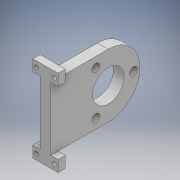
# Autodesk Inventor part: Slipring_mount
Saved by Autodesk Inventor 2017 (Build 210142000, 142)
## iProperties
Created: 2017-04-29
Part Number: Slipring_mount
Material: Generic
Document SubType Name: Modeling
Designer: s4321966
Density: 1 g/cm^3
Appearance: Default
Author: s4321966
Autodesk Inventor part; units mm, degrees
ref_plane "YZ Plane" through (0, 0, 0) normal (1, 0, 0) x (0, 1, 0)
ref_plane "XZ Plane" through (0, 0, 0) normal (0, 1, 0) x (-1, 0, 0)
ref_plane "XY Plane" through (0, 0, 0) normal (0, 0, 1) x (1, 0, 0)
sketch "Sketch1" plane through (0, 0, 0) normal (1, 0, 0) x (0, 1, 0)
  circle A0 centre (0, 0) radius 11
  circle A1 centre (0, 0) radius 22
  circle A2 centre (0, 0) radius 17.5
  circle A3 centre (17.5, 0) radius 2.75
  circle A4 centre (-8.75, 15.1554) radius 2.75
  circle A5 centre (-8.75, -15.1554) radius 2.75
  dimension "d2" = 35
  dimension "d0" = 22
  dimension "d1" = 44
  dimension "d3" = 5.5
  dimension "d6" = 360
  constraints: 5 centre point, 3 coincident, 1 horizontal alignment, 9 other
  measures "d0" diameter of A0
  measures "d1" diameter of A1
  measures "d3" diameter of A3
extrude "Extrusion1" add sketch "Sketch1" along normal blind 7.5 contours A1 | A3 A2 A5 A4
sketch "Sketch2" plane through (7.5, 0, 0) normal (1, 0, 0) x (0, 0, -1)
  arc A0 (2.7415, 17.2839) -> (-2.7415, 17.2839) centre (0, 0) ccw projected
  circle A1 centre (0, 0) radius 17.5
  circle A2 centre (0, 17.5) radius 2.75
  circle A3 centre (-15.1554, -8.75) radius 2.75
  circle A4 centre (15.1554, -8.75) radius 2.75
  dimension "d10" = 35
  dimension "d11" = 5.5
  dimension "d14" = 360
  constraints: 3 centre point, 1 coincident, 1 vertical alignment, 9 other
  measures "d11" diameter of A2
extrude "Extrusion2" cut sketch "Sketch2" against normal blind 10 contours A2 A0 | A0 A2 | A3 A1 | A1 A3 | A4 A1 | A1 A4
sketch "Sketch3" plane through (7.5, 0, 0) normal (1, 0, 0) x (0, 0, -1)
  line L0 (0, 0) -> (0, -40)
  line L1 (0, 0) -> (40, 0) construction
  line L2 (0, -40) -> (50, -40)
  line L3 (0, -40) -> (25, -40)
  line L4 (25, -40) -> (25, -35)
  line L5 (25, -35) -> (0, -35)
  line L6 (0, -35) -> (0, -40)
  line L7 (0, -35) -> (30, -35)
  line L8 (30, -35) -> (30, -40)
  line L9 (30, -40) -> (0, -40)
  line L10 (0, -40) -> (0, -35)
  line L11 (30, -40) -> (-30, -40)
  line L12 (-30, -40) -> (-30, -35)
  line L13 (-30, -35) -> (30, -35)
  line L14 (30, -35) -> (30, -40)
  circle A0 centre (0, 0) radius 22 projected
  line L15 (25, -40) -> (-22, -40)
  line L16 (-22, -40) -> (-22, 0)
  line L17 (-22, 0) -> (25, 0)
  line L18 (22, 0) -> (-22, 0)
  line L19 (-22, 0) -> (-22, -40)
  line L20 (-22, -40) -> (22, -40)
  line L21 (22, -40) -> (22, 0)
  line L22 (30, -35) -> (22, -35)
  line L23 (22, -35) -> (22, -40)
  line L24 (22, -40) -> (30, -40)
  line L25 (30, -40) -> (30, -35)
  line L26 (-30, -35) -> (-22, -35)
  line L27 (-22, -35) -> (-22, -40)
  line L28 (-22, -40) -> (-30, -40)
  line L29 (-30, -40) -> (-30, -35)
  dimension "d18" = 40
  dimension "d19" = 90
  dimension "d20" = 50
  dimension "d21" = 25
  dimension "d22" = 5
  dimension "d23" = 30
  dimension "d24" = 5
  dimension "d25" = 60
  dimension "d26" = 5
  constraints: 60 end point, 13 parallel, 9 perpendicular, 8 horizontal, 2 point on circle, 1 point on line, 1 vertical
  measures "d18" distance of L0.start L0.end
  measures "d19" angle of L0 L1
  measures "d20" distance of L0.end L2.end
  measures "d21" distance of L5.end L4.end
  measures "d22" distance of L4.end L3.end
  measures "d23" distance of L8.end L9.end
  measures "d24" distance of L7.end L8.end
  measures "d25" distance of L12.end L13.end
  measures "d26" distance of L11.end L12.end
extrude "Extrusion3" add sketch "Sketch3" against normal blind 7.5 contours L5 L21 L2 L0 | L13 L16 A0 L0 | L0 A0 L21 L5 | L0 L11 L16 L13 | L5 L4 L2 L21 | L16 L11 L12 L13 | L7 L8 L2 L4
sketch "Sketch5" plane through (7.5, 0, 0) normal (1, 0, 0) x (0, 0, -1)
  line L0 (30, -35) -> (30, -40) projected
  line L1 (22, -35) -> (30, -35) projected
  line L2 (30, -40) -> (22, -40)
  line L3 (22, -40) -> (22, -35)
  line L4 (22, -35) -> (30, -35)
  line L5 (30, -35) -> (30, -40)
  line L6 (-30, -35) -> (-30, -40) projected
  line L7 (-30, -40) -> (-22, -40)
  line L8 (-22, -40) -> (-22, -35)
  line L9 (-22, -35) -> (-30, -35)
  line L10 (-30, -35) -> (-30, -40)
  point P0 (0, 0)
  constraints: 16 end point, 4 parallel, 2 horizontal, 2 perpendicular
extrude "Extrusion5" add sketch "Sketch5" along normal blind 5 and the other way blind 12.5
sketch "Sketch6" plane through (-5, -35, -30) normal (0, 1, 0) x (1, 0, 0)
  line L0 (0, -8) -> (5, -8) projected
  line L1 (0, 0) -> (17.5, 0) projected
  line L2 (5, -8) -> (0, 0)
  line L3 (0, 0) -> (17.5, 0)
  line L4 (12.5, -8) -> (5, -8) projected
  line L5 (17.5, 0) -> (12.5, -8)
  line L6 (0, -52) -> (5, -52) projected
  line L7 (12.5, -8) -> (5, -52)
  line L8 (17.5, -60) -> (0, -60) projected
  line L9 (5, -52) -> (0, -60)
  line L10 (0, -60) -> (17.5, -60)
  line L11 (17.5, -60) -> (12.5, -52)
  circle A0 centre (2.5, -4) radius 1.5
  circle A1 centre (15, -4) radius 1.5
  circle A2 centre (2.5, -56) radius 1.5
  circle A3 centre (15, -56) radius 1.5
  point P0 (5, -30)
  dimension "d45" = 3
  dimension "d46" = 3
  dimension "d47" = 3
  dimension "d48" = 3
  constraints: 14 end point, 4 centre point, 4 equal length, 4 midpoint
  measures "d45" diameter of A0
  measures "d46" diameter of A1
  measures "d47" diameter of A2
  measures "d48" diameter of A3
extrude "Extrusion6" cut sketch "Sketch6" against normal blind 5 contours A0 L2 | L2 A0 | A1 L5 | L5 A1 | A2 L9 | L9 A2 | A3 L11 | L11 A3
body "Solid1"
